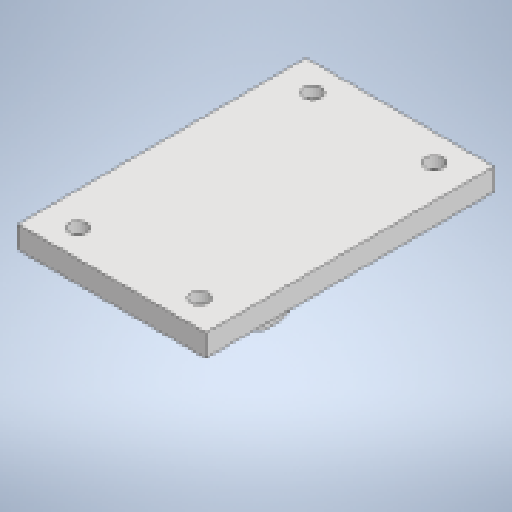
# Autodesk Inventor part: encaixeDuplo
Saved by Autodesk Inventor 2023 (Build 270158000, 158)
## iProperties
Created: 2024-04-11
Part Number: encaixeDuplo
Material: Generic
Document SubType Name: Modeling
Designer: cvss2
Density: 1 g/cm^3
Appearance: Default
Author: cvss2
Autodesk Inventor part; units mm, degrees
ref_plane "YZ Plane" through (0, 0, 0) normal (1, 0, 0) x (0, 1, 0)
ref_plane "XZ Plane" through (0, 0, 0) normal (0, 1, 0) x (-1, 0, 0)
ref_plane "XY Plane" through (0, 0, 0) normal (0, 0, 1) x (1, 0, 0)
sketch "Sketch1" plane through (0, 0, 0) normal (0, 1, 0) x (-1, 0, 0)
  line L0 (0, 0) -> (34, 0)
  line L1 (34, 0) -> (34, -52.1)
  line L2 (34, -52.1) -> (0, -52.1)
  line L3 (0, -52.1) -> (0, 0)
  circle A0 centre (28, -4.85) radius 1.6
  line L4 (28, -8.0832) -> (25.2, -6.4666)
  line L5 (25.2, -6.4666) -> (25.2, -3.2334)
  line L6 (25.2, -3.2334) -> (28, -1.6168)
  line L7 (28, -1.6168) -> (30.8, -3.2334)
  line L8 (30.8, -3.2334) -> (30.8, -6.4666)
  line L9 (30.8, -6.4666) -> (28, -8.0832)
  line L10 (17, 0) -> (17, -52.1) construction
  line L11 (0, -26.05) -> (34, -26.05) construction
  line L12 (17, -19.8) -> (14, -19.8)
  line L13 (14, -19.8) -> (14, -32.3)
  line L14 (14, -32.3) -> (17, -32.3)
  line L15 (17, -32.3) -> (17, -19.8)
  line L16 (23.2, -19.8) -> (20.2, -19.8)
  line L17 (20.2, -19.8) -> (20.2, -32.3)
  line L18 (20.2, -32.3) -> (23.2, -32.3)
  line L19 (23.2, -32.3) -> (23.2, -19.8)
  dimension "d0" = 34
  dimension "d1" = 52.1
  dimension "d2" = 3.2
  dimension "d3" = 4.85
  dimension "d4" = 6
  dimension "d5" = 5.6
  dimension "d18" = 3
  dimension "d19" = 12.5
  dimension "d20" = 3
  dimension "d21" = 12.5
  dimension "d22" = 19.8
  dimension "d23" = 3.2
  constraints: 40 end point, 6 parallel, 4 midpoint, 3 horizontal, 3 perpendicular, 2 point on line, 1 centre point, 1 coincident, 13 other
  measures "d0" distance of L1.end L2.end
  measures "d1" distance of L0.end L1.end
  measures "d2" diameter of A0
  measures "d3" distance from line of L0 A0.centre
  measures "d4" distance from line of L1 A0.centre
  measures "d5" distance between parallel lines of L8 L5
  measures "d18" distance of L14.end L13.end
  measures "d19" distance of L13.end L12.end
  measures "d20" distance of L18.end L17.end
  measures "d21" distance of L17.end L16.end
  measures "d22" distance between parallel lines of L2 L14
  measures "d23" distance between parallel lines of L15 L17
extrude "Extrusion1" add sketch "Sketch1" along normal blind 4 contours L0 L1 L2 L3 | A0 | L4 L5 L6 L7 L8 L9 | L15 L14 L13 L12 | L19 L18 L17 L16
extrude "Extrusion2" cut sketch "Sketch1" along normal blind 2 contours L4 L5 L6 L7 L8 L9
extrude "Extrusion3" cut sketch "Sketch1" along normal blind 4 contours A0
pattern_linear "Rectangular Pattern1" count 2 spacing 42.4 along (0, 0, -1) count 2 spacing 22 along (1, 0, 0) of "Extrusion3", "Extrusion2"
extrude "Extrusion4" add sketch "Sketch1" against normal blind 15 contours L15 L14 L13 L12 | L19 L18 L17 L16
sketch "Sketch2" plane through (-14, -15, -19.8) normal (1, 0, 0) x (0, 0, -1)
  line L0 (0, 15) -> (12.5, 15) projected
  line L1 (0, 15) -> (0, 0) projected
  line L2 (12.5, 0) -> (0, 0) projected
  line L3 (12.5, 15) -> (12.5, 0) projected
  circle A0 centre (6.25, 6.25) radius 1.65
  point P0 (-19.8, 15)
  dimension "d26" = 3.3
  dimension "d27" = 12.5
  dimension "d28" = 6.25
  dimension "d29" = 6.25
  constraints: 1 centre point
  measures "d26" diameter of A0
  measures "d27" distance of L2.start L1.end
  measures "d28" distance from line of L2 A0.centre
  measures "d29" distance from line of L3 A0.centre
extrude "Extrusion5" cut sketch "Sketch2" against normal up to surface (9.2 mm away) contours A0
fillet "Fillet1" radius 6.25 4 edges at (-15.5, -15, -19.8) (-15.5, -15, -32.3) (-21.7, -15, -19.8) (-21.7, -15, -32.3)
fillet "Fillet2" radius 4 4 edges at (-15.5, 0, -19.8) (-15.5, 0, -32.3) (-21.7, 0, -19.8) (-21.7, 0, -32.3)
equation "\"d22\" = -0.5 * d19 + 0.5 * d1"
equation "\"d28\" = 0.5 * d27"
equation "\"d29\" = d28"
body "Solid1"
